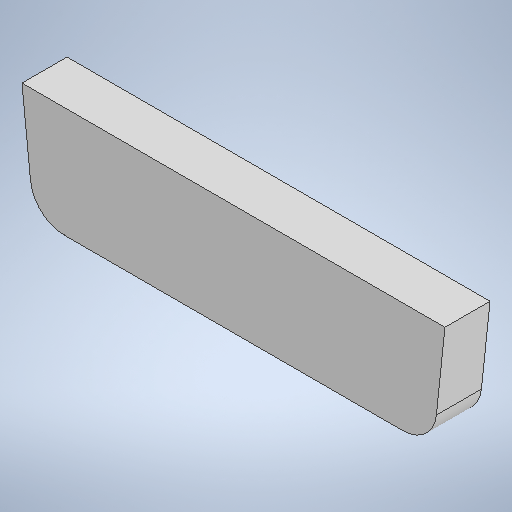
# Autodesk Inventor part: Divider_Short
Saved by Autodesk Inventor 2025 (Build 290162010, 162A)
## iProperties
Created: 2024-09-20
Part Number: Divider_Short
Material: Generic
Document SubType Name: Modeling
Designer: vncnt
Density: 1 g/cm^3
Appearance: Default
Author: vncnt
## iProperties of the stored document Divider_3DPrint.ipt
Created: 2024-09-20
Part Number: Divider_3DPrint
Material: Generic
Document SubType Name: Modeling
Designer: vncnt
Density: 1 g/cm^3
Appearance: Default
Author: vncnt
Autodesk Inventor part; units mm, degrees
ref_plane "YZ Plane" through (0, 0, 0) normal (1, 0, 0) x (0, 1, 0)
ref_plane "XZ Plane" through (0, 0, 0) normal (0, 1, 0) x (-1, 0, 0)
ref_plane "XY Plane" through (0, 0, 0) normal (0, 0, 1) x (1, 0, 0)
sketch "Sketch1" plane through (0, 0, 0) normal (0, 0, 1) x (1, 0, 0)
  line L0 (17.1248, 0) -> (207.8752, 0)
  line L1 (-6.65, 62.3) -> (231.65, 62.3)
  line L2 (-6.65, 62.3) -> (-1.8176, 17.0281)
  line L3 (226.8176, 17.0281) -> (231.65, 62.3)
  arc A0 (-1.8176, 17.0281) -> (17.1248, 0) centre (17.1248, 19.05) ccw
  arc A1 (207.8752, 0) -> (226.8176, 17.0281) centre (207.8752, 19.05) ccw
  point P0 (0, 0)
  point P1 (225, 0)
  point P2 (112.5, 0)
  point P3 (112.5, 62.3)
  dimension "d0" = 225
  dimension "d1" = 62.3
  dimension "d2" = 238.3
  dimension "d4" = 19.05
  dimension "d11" = 0
  constraints: 8 end point, 4 point on circle, 4 point on line, 4 tangent, 2 centre point, 2 midpoint, 1 equal radius, 1 horizontal, 1 parallel
  measures "d0" distance of point (0, 0) point (225, 0)
  measures "d1" distance between parallel lines of L0 L1
  measures "d2" distance of L1.start L1.end
  measures "d4" radius of A0
  measures "d11" horizontal distance of point (112.5, 0) point (112.5, 62.3)
extrude "Extrusion1" add sketch "Sketch1" along normal blind 25.4
sketch "Sketch2" plane through (0, 0, 25.4) normal (0, 0, 1) x (1, 0, 0)
  line L0 (243.0343, 163.5066) -> (27.3006, 163.5066)
  line L1 (27.3006, 163.5066) -> (27.3006, 18.9917)
  line L2 (27.3006, 18.9917) -> (243.0343, 18.9917)
  line L3 (243.0343, 18.9917) -> (243.0343, 163.5066)
  line L4 (27.1522, 18.9917) -> (243.0343, 18.9917)
  line L5 (243.0343, 18.9917) -> (243.0343, -17.0628)
  line L6 (243.0343, -17.0628) -> (27.1522, -17.0628)
  line L7 (27.1522, -17.0628) -> (27.1522, 18.9917)
  point P0 (0, 0)
  constraints: 16 end point, 4 parallel, 2 horizontal, 2 perpendicular, 1 point on line
extrude "Test" [suppressed]
body "Solid1"
